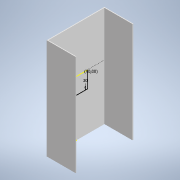
# Autodesk Inventor part: Caja
Saved by Autodesk Inventor 2021 (Build 250183000, 183)
## iProperties
Created: 2022-11-24
Part Number: Caja
Material: Genérico
Document SubType Name: Modeling
Designer: sergi
Density: 1 g/cm^3
Appearance: Valor por defecto
Author: sergi
Autodesk Inventor part; units mm, degrees
ref_plane "YZ Plane" through (0, 0, 0) normal (1, 0, 0) x (0, 1, 0)
ref_plane "XZ Plane" through (0, 0, 0) normal (0, 1, 0) x (-1, 0, 0)
ref_plane "XY Plane" through (0, 0, 0) normal (0, 0, 1) x (1, 0, 0)
sketch "Boceto1" plane through (0, 0, 0) normal (0, 1, 0) x (-1, 0, 0)
  line L0 (-53, -53) -> (53, -53)
  line L1 (53, -53) -> (53, 53)
  line L2 (53, 53) -> (-53, 53)
  line L3 (-53, 53) -> (-53, -53)
  line L4 (-53, -53) -> (53, 53) construction
  line L5 (53, -53) -> (-53, 53) construction
  point P0 (0, 0)
  dimension "d0" = 106
  dimension "d1" = 106
  constraints: 12 end point, 2 midpoint, 2 parallel, 1 horizontal, 1 perpendicular
  measures "d0" distance of L2.end L1.end
  measures "d1" distance of L1.end L0.end
extrude "Extrusión1" add sketch "Boceto1" along normal blind 185
shell "Vaciado1" thickness 1.5 removed faces 2 at (17.6667, 185, -17.6667) at (17.6667, 0, -17.6667)
split "Dividir1" plane through (0, 0, 0) removes the side toward (1, 0, 0)
sketch "Boceto2" plane through (-51.5, 0, -51.5) normal (1, 0, 0) x (0, 0, -1)
  line L0 (-71.9943, 102) -> (-31.0057, 102) projected
  line L1 (-31.0057, 102) -> (-31.0057, 72)
  line L2 (-31.0057, 102) -> (-1.0057, 102) construction
  line L3 (-31.0057, 72) -> (-71.9943, 72)
  line L4 (-71.9943, 72) -> (-71.9943, 102)
  point P0 (-51.5, 0)
  dimension "d5" = 30
  dimension "d6" = 90
  constraints: 8 end point, 3 perpendicular, 1 horizontal, 1 vertical
  measures "d5" distance of L0.end L1.end
  measures "d6" angle of L1 L2
extrude "Extrusión2" cut sketch "Boceto2" against normal blind 10
